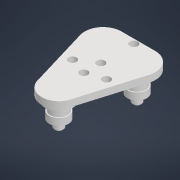
# Autodesk Inventor part: Stationary bracket V2
Saved by Autodesk Inventor 2022 (Build 260153000, 153)
## iProperties
Created: 2022-01-30
Part Number: Stationary bracket V2
Material: Generic
Document SubType Name: Modeling
Designer: izack
Density: 1 g/cm^3
Appearance: Default
Author: izack
## iProperties of the stored document Stationary Bracket_3DPrint.ipt
Part Number: Stationary Bracket_3DPrint
Material: Generic
Document SubType Name: Modeling
Designer: izack
Appearance: Default
Author: izack
Autodesk Inventor part; units mm, degrees
ref_plane "YZ Plane" through (0, 0, 0) normal (1, 0, 0) x (0, 1, 0)
ref_plane "XZ Plane" through (0, 0, 0) normal (0, 1, 0) x (-1, 0, 0)
sketch "Sketch1" plane through (0, 0, 0) normal (0, 1, 0) x (-1, 0, 0)
  line L0 (-7, 10.5) -> (7, 10.5)
  line L1 (7, 10.5) -> (7, -10.5)
  line L2 (7, -10.5) -> (-7, -10.5)
  line L3 (-7, -10.5) -> (-7, 10.5)
  line L4 (-7, 10.5) -> (7, -10.5) construction
  line L5 (7, 10.5) -> (-7, -10.5) construction
  line L6 (-7, 7.5) -> (7, 7.5)
  line L7 (7, 7.5) -> (7, -7.5)
  line L8 (7, -7.5) -> (-7, -7.5)
  line L9 (-7, -7.5) -> (-7, 7.5)
  line L10 (-7, 7.5) -> (7, -7.5) construction
  line L11 (7, 7.5) -> (-7, -7.5) construction
  line L12 (7, 0) -> (-7, 0) construction
  circle A0 centre (3.5, 0) radius 1.25
  circle A1 centre (-3.5, 0) radius 1.25
  point P0 (0, 0)
  dimension "d0" = 14
  dimension "d1" = 21
  dimension "d2" = 15
  dimension "d3" = 2.5
  dimension "d4" = 2.5
  dimension "d5" = 3.5
  dimension "d6" = 3.5
  constraints: 26 end point, 6 midpoint, 4 parallel, 3 point on line, 2 centre point, 2 horizontal, 2 perpendicular
  measures "d0" distance of L1.end L2.end
  measures "d1" distance of L0.end L1.end
  measures "d2" distance of L6.end L7.end
  measures "d3" diameter of A0
  measures "d4" diameter of A1
  measures "d5" distance from line of L1 A0.centre
  measures "d6" distance from line of L3 A1.centre
extrude "Extrusion1" add sketch "Sketch1" along normal blind 3
sketch "Sketch2" plane through (0, 0, 0) normal (0, -1, 0) x (1, 0, 0)
  line L0 (7, -10.5) -> (-7, -10.5) projected
  line L1 (7, 10.5) -> (7, -10.5) projected
  line L2 (-7, -10.5) -> (7, -10.5)
  line L3 (7, -10.5) -> (7, -7.5)
  line L4 (7, -7.5) -> (-7, -7.5)
  line L5 (-7, -7.5) -> (-7, -10.5)
  line L6 (-7, 10.5) -> (7, 10.5) projected
  line L7 (-7, 10.5) -> (7, 10.5)
  line L8 (7, 10.5) -> (7, 7.5)
  line L9 (7, 7.5) -> (-7, 7.5)
  line L10 (-7, 7.5) -> (-7, 10.5)
  point P0 (0, 0)
  dimension "d9" = 3
  dimension "d10" = 3
  constraints: 16 end point, 4 parallel, 2 horizontal, 2 perpendicular, 2 point on line
  measures "d9" distance of L3.end L2.end
  measures "d10" distance of L7.end L8.end
extrude "Extrusion2" add sketch "Sketch2" along normal blind 18
sketch "Sketch3" plane through (-7, 3, 10.5) normal (0, 0, 1) x (1, 0, 0)
  line L0 (14, -3) -> (0, -3) projected
  line L1 (0, -3) -> (14, -3)
  line L2 (0, -3) -> (0, -21) construction
  line L3 (0, -6.5) -> (14, -6.5) construction
  circle A0 centre (7, -13.5) radius 1.75
  circle A1 centre (7, -6.5) radius 1.75
  line L4 (14, -21) -> (14, 0) projected
  line L5 (7, -3) -> (7, -16.789) construction
  dimension "d14" = 3.5
  dimension "d15" = 3.5
  dimension "d32" = 3.5
  dimension "d33" = 7
  constraints: 6 end point, 3 point on line, 2 centre point, 1 collinear, 1 horizontal, 1 midpoint, 1 vertical
  measures "d14" diameter of A0
  measures "d15" diameter of A1
  measures "d32" distance from line of A1.centre L0
  measures "d33" distance of A1.centre A0.centre
extrude "Extrusion3" cut sketch "Sketch3" against normal through all
sketch "Sketch4" plane through (-7, 0, -7.5) normal (0, 0, 1) x (1, 0, 0)
  line L0 (0, 0) -> (0, -18) projected
  line L1 (14, 0) -> (14, -18) projected
  line L2 (0, -18) -> (14, -18)
  line L3 (14, -18) -> (14, -15)
  line L4 (14, -15) -> (0, -15)
  line L5 (0, -15) -> (0, -18)
  point P0 (7, 0)
  point P1 (0, -15)
  dimension "d20" = 3
  constraints: 8 end point, 2 parallel, 1 horizontal, 1 perpendicular, 1 point on line
  measures "d20" distance of L3.end L2.end
extrude "Extrusion4" add sketch "Sketch4" along normal up to surface (15 mm away)
sketch "Sketch5" plane through (0, -18, 0) normal (0, -1, 0) x (1, 0, 0)
  circle A0 centre (7.5, -13.5) radius 3.85
  circle A1 centre (0, 13.5) radius 3.85
  line L0 (7, 10.5) -> (-7, 10.5) projected
  line L1 (-7, -10.5) -> (7, -10.5) projected
  line L2 (-7, 10.5) -> (-7, -10.5) projected
  line L3 (-7, 10.5) -> (7, 10.5)
  line L4 (-7, -10.5) -> (7, -10.5)
  line L5 (-1.75, 10.5) -> (1.75, 10.5) construction
  line L6 (0, 10.5) -> (0, -10.5) construction
  line L7 (7, -10.5) -> (-7, -10.5) construction
  circle A2 centre (-7.5, -13.5) radius 3.85
  line L8 (-7, 10.5) -> (7, 10.5) projected
  circle A3 centre (0, 13.5) radius 7.6158
  circle A4 centre (7.5, -13.5) radius 8.0777
  circle A5 centre (-7.5, -13.5) radius 8.0777
  line L9 (-7.5, 14.8229) -> (-15.2423, -11.1962)
  line L10 (-7.5, -21.5777) -> (7.5, -21.5777)
  line L11 (15.2423, -11.1962) -> (7.5, 14.8229)
  point P0 (0, 0)
  point P1 (-7, -7.5)
  point P2 (-7, 7.5)
  point P3 (0, -13.5)
  point P4 (3.65, -13.5)
  point P5 (-3.85, 13.5)
  point P6 (-11.3217, -13.9658)
  point P7 (0, -16.5)
  point P8 (-2.413, 10.5)
  point P9 (2.413, 10.5)
  point P10 (-7, -9.6826)
  point P11 (-5.087, -10.5)
  dimension "d23" = 7.7
  dimension "d24" = 7.7
  dimension "d35" = 7.7
  dimension "d25" = 6
  dimension "d26" = 6
  dimension "d34" = 7.5
  dimension "d36" = 7.5
  dimension "d37" = 6
  constraints: 12 end point, 9 point on circle, 4 coincident, 3 centre point, 2 equal length, 2 midpoint, 2 tangent, 1 horizontal, 1 horizontal alignment, 8 other
  measures "d25" vertical distance of point (-7, -7.5) point (7.5, -13.5)
  measures "d26" vertical distance of point (0, 13.5) point (-7, 7.5)
  measures "d34" distance from line of L6 point (7.5, -13.5)
  measures "d36" distance from line of L6 point (-7.5, -13.5)
  measures "d37" vertical distance of point (-7, -7.5) point (-7.5, -13.5)
extrude "Extrusion5" add sketch "Sketch5" against normal blind 3 contours A1 L0 A3 | A1 L0 A3 | A3 L11 A4 A5 L2 | L2 A5 L9 A3 | A5 L1 A2 L2 | L2 A2 L1 A4 A5 | A5 A4 | A4 A5 | A4 L10 A5
sketch "Sketch6" plane through (0, 3, 0) normal (0, 1, 0) x (1, 0, 0)
  line L0 (-7, 10.5) -> (-7, -10.5) projected
  line L1 (-7, -10.5) -> (7, -10.5) projected
  line L2 (-7, -10.5) -> (7, -10.5) projected
  line L3 (7, -10.5) -> (7, 10.5) projected
  line L4 (7, 10.5) -> (-7, 10.5) projected
  line L5 (-7, 10.5) -> (-7, -10.5) projected
  circle A0 centre (3.5, 0) radius 1.25 projected
  circle A1 centre (-3.5, 0) radius 1.25 projected
  point P0 (0, 0)
extrude "Extrusion6" cut sketch "Sketch6" against normal up to surface (3 mm away)
fillet "Fillet1" radius 2 4 edges at (-7, 0, -9) (7, 0, -9) (-7, 0, 9) (7, 0, 9)
extrude "Extrusion7" add sketch "Sketch5" along normal blind 17.8 and the other way blind 3 contours A0 | A1 L0 | L0 A1 | A2 L1 L2 | L2 L1 A2
sketch "Sketch8" plane through (0, -18, 0) normal (0, -1, 0) x (1, 0, 0)
  circle A0 centre (0, 13.5) radius 3.85 projected
  circle A1 centre (-7.5, -13.5) radius 3.85 projected
  circle A2 centre (7.5, -13.5) radius 3.85 projected
  circle A3 centre (7.5, -13.5) radius 6
  circle A4 centre (0, 13.5) radius 6
  circle A5 centre (-7.5, -13.5) radius 6
  point P0 (0, 0)
  dimension "d44" = 12
  dimension "d45" = 12
  dimension "d46" = 12
  constraints: 3 centre point, 3 coincident
  measures "d44" diameter of A3
  measures "d45" diameter of A4
  measures "d46" diameter of A5
extrude "Extrusion9" add sketch "Sketch8" along normal blind 2
sketch "Sketch9" plane through (0, -35.8, 13.5) normal (0, -1, 0) x (1, 0, 0)
  circle A0 centre (7.5, -27) radius 6 projected
  circle A1 centre (-7.5, -27) radius 6 projected
  circle A2 centre (0, 0) radius 6 projected
  point P0 (0, -13.5)
extrude "Extrusion10" add sketch "Sketch9" against normal blind 2
sketch "Sketch10" plane through (0, -35.8, 13.5) normal (0, -1, 0) x (1, 0, 0)
  circle A0 centre (0, 0) radius 6 projected
  circle A1 centre (7.5, -27) radius 6 projected
  circle A2 centre (-7.5, -27) radius 6 projected
  line L0 (-7.5, -35.0777) -> (7.5, -35.0777) projected
  arc A3 (7.5, -35.0777) -> (15.2423, -24.6962) centre (7.5, -27) ccw projected
  line L1 (15.2423, -24.6962) -> (7.5, 1.3229) projected
  arc A4 (7.5, 1.3229) -> (-7.5, 1.3229) centre (0, 0) ccw projected
  line L2 (-7.5, 1.3229) -> (-15.2423, -24.6962) projected
  arc A5 (-15.2423, -24.6962) -> (-7.5, -35.0777) centre (-7.5, -27) ccw projected
  circle A6 centre (0, 0) radius 6 projected
  circle A7 centre (-7.5, -27) radius 3.85 projected
  circle A8 centre (-7.5, -27) radius 6 projected
  circle A9 centre (7.5, -27) radius 3.85 projected
  circle A10 centre (7.5, -27) radius 6 projected
  point P0 (0, -13.5)
extrude "Extrusion11" add sketch "Sketch10" along normal blind 3 contours A0 | A1 | A2 | A5 L2 A4 L1 A3 L0 | A7 | A9
ref_plane "Work Plane1" through (0, -26.9, 13.5) normal (0, 1, 0) x (1, 0, 0)
split "Split1" plane through (0, -26.9, 13.5) removes the side toward (0, -1, 0)
sketch "Sketch11" plane through (0, -26.9, 13.5) normal (0, 1, 0) x (1, 0, 0)
  circle A0 centre (0, 0) radius 3.85 projected
  circle A1 centre (0, 0) radius 2
  circle A2 centre (0, 0) radius 4.25
  circle A3 centre (7.5, 27) radius 3.85 projected
  circle A4 centre (-7.5, 27) radius 3.85 projected
  circle A5 centre (7.5, 27) radius 2
  circle A6 centre (-7.5, 27) radius 2
  circle A7 centre (7.5, 27) radius 4.25
  circle A8 centre (-7.5, 27) radius 4.25
  point P0 (0, 13.5)
  dimension "d53" = 4
  dimension "d54" = 8.5
  dimension "d57" = 4
  dimension "d58" = 4
  dimension "d62" = 8.5
  dimension "d63" = 8.5
  constraints: 6 centre point, 6 coincident
  measures "d53" diameter of A1
  measures "d54" diameter of A2
  measures "d57" diameter of A5
  measures "d58" diameter of A6
  measures "d62" diameter of A7
  measures "d63" diameter of A8
extrude "Extrusion12" add sketch "Sketch11" against normal blind 4 contours A1 | A5 | A6
chamfer "Chamfer1" distance 0.75 angle 45 3 edges at (5.5, -30.9, -13.5) (-9.5, -30.9, -13.5) (-2, -30.9, 13.5)
extrude "Extrusion13" add sketch "Sketch11" along normal blind 3.1 contours A0 | A1 | A2 | A3 | A4 | A5 | A6 | A7 | A8
sketch "Sketch12" plane through (-5, 0, 7.5) normal (0, 1, 0) x (1, 0, 0)
  line L0 (17.1671, -5.9005) -> (-16.9008, -5.9005)
  line L1 (-16.9008, -5.9005) -> (-16.9008, 22.3006)
  line L2 (-16.9008, 22.3006) -> (17.1671, 22.3006)
  line L3 (17.1671, 22.3006) -> (17.1671, -5.9005)
  point P0 (5, 7.5)
  constraints: 8 end point, 2 parallel, 1 horizontal, 1 perpendicular
extrude "Extrusion14" cut sketch "Sketch12" against normal up to surface (15 mm away)
sketch "Sketch13" plane through (0, -15, 13.5) normal (0, 1, 0) x (1, 0, 0)
  line L0 (7.5, 35.0777) -> (-7.5, 35.0777) construction
  line L1 (0, 35.0777) -> (0, -7.6158) construction
  arc A0 (-7.5, -1.3229) -> (7.5, -1.3229) centre (0, 0) ccw construction
  line L2 (15.2423, 24.6962) -> (7.5, -1.3229) construction
  line L3 (-7.5, -1.3229) -> (-15.2423, 24.6962) construction
  circle A1 centre (0, 33.0799) radius 1.75
  circle A2 centre (0, 11) radius 1.75
  circle A3 centre (7.5, 13.5) radius 1.75
  circle A4 centre (-7.5, 13.5) radius 1.75
  circle A5 centre (-7.5, 27) radius 6 construction
  circle A6 centre (7.5, 27) radius 6 construction
  circle A7 centre (0, 0) radius 6 construction
  circle A8 centre (0, 18.5) radius 1.75
  point P0 (0, 13.5)
  dimension "d68" = 3.5
  dimension "d69" = 3.5
  dimension "d70" = 3.5
  dimension "d71" = 3.5
  dimension "d73" = 13.5
  dimension "d74" = 13.5
  dimension "d75" = 11
  dimension "d78" = 7.5
  dimension "d79" = 7.5
  dimension "d80" = 3.5
  dimension "d81" = 7.5
  constraints: 5 centre point, 3 point on line, 2 end point, 1 midpoint, 1 point on circle, 1 vertical
  measures "d68" diameter of A1
  measures "d69" diameter of A2
  measures "d70" diameter of A3
  measures "d71" diameter of A4
  measures "d73" vertical distance of A0.centre A3.centre
  measures "d74" vertical distance of A0.centre A4.centre
  measures "d75" distance of A0.centre A2.centre
  measures "d78" distance from line of L1 A4.centre
  measures "d79" distance from line of L1 A3.centre
  measures "d80" diameter of A8
  measures "d81" distance of A2.centre A8.centre
extrude "Extrusion15" cut sketch "Sketch13" against normal blind 3.5
equation "\"d76\" = d69"
body "Solid1"
